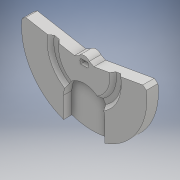
# Autodesk Inventor part: RescueKitThrow-Joint
Saved by Autodesk Inventor 2018.3 (Build 223284000, 284)
## iProperties
Created: 2019-02-13
Part Number: RescueKitThrow-Joint
Material: 一般
Document SubType Name: Modeling
Designer: TOMOKI
Density: 1 g/cm^3
Appearance: 既定
Author: TOMOKI
Autodesk Inventor part; units mm, degrees
note: some values were not read from the file. Chosen so that the rebuilt part matches the saved one: sketch regions of "押し出し9".
ref_plane "YZ Plane" through (0, 0, 0) normal (1, 0, 0) x (0, 1, 0)
ref_plane "XZ Plane" through (0, 0, 0) normal (0, 1, 0) x (-1, 0, 0)
ref_plane "XY Plane" through (0, 0, 0) normal (0, 0, 1) x (1, 0, 0)
sketch "スケッチ1" plane through (0, 0, 0) normal (0, 1, 0) x (-1, 0, 0)
  arc A0 (54.8142, 37.6946) -> (46.9358, 37.6946) centre (50.875, 37) ccw
  circle A1 centre (50.875, 13.875) radius 12.5
  line L0 (50.875, 37) -> (87.3129, 43.425)
  line L1 (50.875, 37) -> (87.875, 37) construction
  line L2 (87.3129, 43.425) -> (50.875, 37)
  line L3 (50.875, 37) -> (14.4371, 43.425)
  arc A2 (13.4523, 43.5986) -> (88.2977, 43.5986) centre (50.875, 37) ccw
  line L4 (87.3129, 43.425) -> (88.2977, 43.5986)
  line L5 (13.4523, 43.5986) -> (14.4371, 43.425)
  point P0 (0, 0)
  dimension "d22" = 25
  dimension "d27" = 10
  dimension "d38" = 4
  dimension "d49" = 76
  constraints: 12 end point, 4 point on circle, 3 centre point, 2 coincident, 2 point on line, 1 collinear, 1 equal length, 1 horizontal
  measures "d22" diameter of A1
  measures "d27" angle of L1 L0
  measures "d38" radius of A0
  measures "d49" diameter of A2
extrude "押し出し1" add sketch "スケッチ1" along normal blind 7
sketch "スケッチ2" plane through (0, 7, 0) normal (0, 1, 0) x (1, 0, 0)
  circle A0 centre (-50.875, -13.875) radius 12.5
  circle A1 centre (-50.875, -13.875) radius 12.5
  point P0 (0, 0)
  constraints: 2 centre point, 2 coincident, 1 concentric
extrude "押し出し2" add sketch "スケッチ2" against normal blind 2
sketch "スケッチ3" plane through (0, 0, 0) normal (0, -1, 0) x (1, 0, 0)
  circle A0 centre (-50.875, 13.875) radius 12.5 projected
  circle A1 centre (-50.875, 13.875) radius 12.5 projected
  line L0 (-63.375, 13.875) -> (-38.375, 13.875)
  line L1 (-38.375, 13.875) -> (-38.375, -3.3785)
  line L2 (-38.375, -3.3785) -> (-63.375, -3.3785)
  line L3 (-63.375, -3.3785) -> (-63.375, 13.875)
  line L4 (-46.9358, 37.6946) -> (-13.4523, 43.5986) projected
  line L5 (-88.2977, 43.5986) -> (-54.8142, 37.6946) projected
  arc A2 (-88.2977, 43.5986) -> (-13.4523, 43.5986) centre (-50.875, 37) ccw projected
  arc A3 (-46.9358, 37.6946) -> (-54.8142, 37.6946) centre (-50.875, 37) ccw projected
  point P0 (0, 0)
  constraints: 8 end point, 2 parallel, 1 horizontal, 1 horizontal alignment, 1 perpendicular, 1 other
extrude "押し出し3" cut sketch "スケッチ3" against normal blind 5 contours L1 A2 L3 A0 | A0 L0 | L1 L2 L3 A2 picked at (-53.2419, 10.4459)
sketch "スケッチ4" plane through (0, 0, 0) normal (0, -1, 0) x (1, 0, 0)
  circle A0 centre (-50.875, 37) radius 2.6
  arc A1 (-38.375, 13.875) -> (-63.375, 13.875) centre (-50.875, 13.875) ccw projected
  line L0 (-63.375, 1.1148) -> (-63.375, 13.875) projected
  line L1 (-38.375, 13.875) -> (-38.375, 1.1148) projected
  line L2 (-46.9358, 37.6946) -> (-13.4523, 43.5986) projected
  line L3 (-52.9987, 38.5) -> (-48.7513, 38.5)
  line L4 (-42.875, 38.5) -> (-42.875, 38.4106)
  line L5 (-48.7513, 35.5) -> (-52.9987, 35.5)
  line L6 (-58.875, 38.4106) -> (-58.875, 38.5)
  arc A2 (-38.375, 1.1148) -> (-13.4523, 43.5986) centre (-50.875, 37) ccw projected
  line L7 (-88.2977, 43.5986) -> (-54.8142, 37.6946) projected
  arc A3 (-88.2977, 43.5986) -> (-63.375, 1.1148) centre (-50.875, 37) ccw projected
  arc A4 (-46.9358, 37.6946) -> (-54.8142, 37.6946) centre (-50.875, 37) ccw projected
  point P0 (0, 0)
  dimension "d12" = 5.2
  dimension "d47" = 3
  constraints: 8 end point, 4 point on circle, 2 parallel, 1 centre point, 1 horizontal, 1 perpendicular, 1 point on line
  measures "d12" diameter of A0
  measures "d47" distance between parallel lines of L5 L3
extrude "押し出し4" cut sketch "スケッチ4" against normal blind 8 contours A0 L5 L3
chamfer "面取り1" distance 2 angle 45 4 edges at (-88.2977, 3.5, 43.5986) (-46.9358, 3.5, 37.6946) (-13.4523, 3.5, 43.5986) (-54.8142, 3.5, 37.6946)
sketch "スケッチ8" plane through (0, 7, 0) normal (0, 1, 0) x (1, 0, 0)
  line L0 (-44.9662, -38.0419) -> (-15.4219, -43.2513) projected
  arc A0 (-48.7513, -38.5) -> (-48.7513, -35.5) centre (-50.875, -37) ccw projected
  arc A1 (-13.157, -41.6206) -> (-88.593, -41.6206) centre (-50.875, -37) ccw projected
  line L1 (-86.3281, -43.2513) -> (-56.7838, -38.0419) projected
  arc A2 (-52.9987, -35.5) -> (-52.9987, -38.5) centre (-50.875, -37) ccw projected
  line L2 (-52.9987, -35.5) -> (-48.7513, -35.5) projected
  line L3 (-48.7513, -38.5) -> (-52.9987, -38.5) projected
  arc A3 (-53.9856, -39.5148) -> (-47.7644, -39.5148) centre (-50.875, -37) ccw projected
  line L4 (-13.157, -41.6206) -> (-15.4219, -43.2513) projected
  line L5 (-86.3281, -43.2513) -> (-88.593, -41.6206) projected
  line L6 (-53.9856, -39.5148) -> (-56.7838, -38.0419) projected
  line L7 (-44.9662, -38.0419) -> (-47.7644, -39.5148) projected
  point P0 (0, 0)
extrude "押し出し8" cut sketch "スケッチ8" along normal blind 0.5 contours L3 A2 L2 A0
sketch "スケッチ9" plane through (0, 0, 0) normal (0, -1, 0) x (1, 0, 0)
  line L0 (-48.7513, 35.5) -> (-52.9987, 35.5) projected
  arc A0 (-52.9987, 38.5) -> (-52.9987, 35.5) centre (-50.875, 37) ccw projected
  arc A1 (-48.7513, 35.5) -> (-48.7513, 38.5) centre (-50.875, 37) ccw projected
  line L1 (-44.9662, 38.0419) -> (-15.4219, 43.2513) projected
  line L2 (-63.375, 1.1148) -> (-63.375, 13.875) projected
  arc A2 (-38.375, 13.875) -> (-63.375, 13.875) centre (-50.875, 13.875) ccw projected
  line L3 (-38.375, 13.875) -> (-38.375, 1.1148) projected
  circle A3 centre (-50.875, 37) radius 17.5
  circle A4 centre (-50.875, 37) radius 20.5
  circle A5 centre (-50.875, 37) radius 19
  line L4 (-86.3281, 43.2513) -> (-56.7838, 38.0419) projected
  arc A6 (-88.593, 41.6206) -> (-63.375, 1.1148) centre (-50.875, 37) ccw projected
  arc A7 (-38.375, 1.1148) -> (-13.157, 41.6206) centre (-50.875, 37) ccw projected
  line L5 (-52.9987, 38.5) -> (-48.7513, 38.5) projected
  arc A8 (-47.7644, 39.5148) -> (-53.9856, 39.5148) centre (-50.875, 37) ccw projected
  line L6 (-15.4219, 43.2513) -> (-13.157, 41.6206) projected
  line L7 (-47.7644, 39.5148) -> (-44.9662, 38.0419) projected
  line L8 (-56.7838, 38.0419) -> (-53.9856, 39.5148) projected
  line L9 (-88.593, 41.6206) -> (-86.3281, 43.2513) projected
  point P0 (0, 0)
  dimension "d39" = 35
  dimension "d40" = 41
  dimension "d41" = 38
  constraints: 3 centre point, 2 coincident
  measures "d39" diameter of A3
  measures "d40" diameter of A4
  measures "d41" diameter of A5
extrude "押し出し9" cut sketch "スケッチ9" against normal blind 2 contours L0 A0 L5 A1 | A3 L4 A5 L1 | L1 A5 A2 A3 | A5 L4 A4 L1 | L1 A4 A2 A5 | A3 A2 A5 L4 | A5 A2 A4 L4 | A2 A5 A3 | A2 A4 A5
chamfer "面取り2" distance 2 angle 45 4 edges at (-69.646, 0, 28.7598) (-32.104, 0, 28.7598) (-66.8754, 0, 29.9123) (-34.8746, 0, 29.9123)
